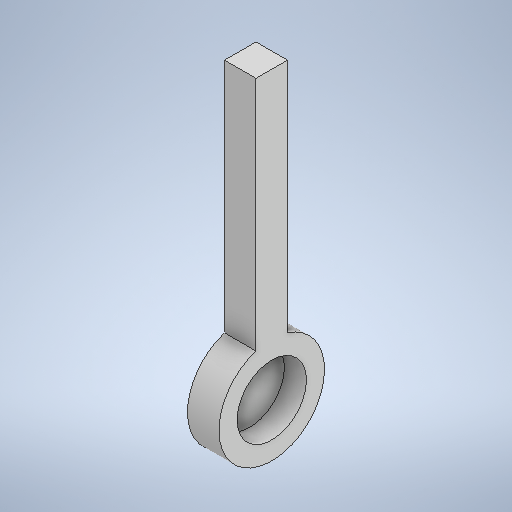
# Autodesk Inventor part: prototype3_2
Saved by Autodesk Inventor 2025.1 (Build 291241020, 241B)
## iProperties
Created: 2024-11-22
Part Number: prototype3_2
Material: Generic
Document SubType Name: Modeling
Designer: leon-
Density: 1 g/cm^3
Appearance: Default
Author: leon-
Autodesk Inventor part; units mm, degrees
ref_plane "YZ Plane" through (0, 0, 0) normal (1, 0, 0) x (0, 1, 0)
ref_plane "XZ Plane" through (0, 0, 0) normal (0, 1, 0) x (-1, 0, 0)
ref_plane "XY Plane" through (0, 0, 0) normal (0, 0, 1) x (1, 0, 0)
sketch "Sketch1" plane through (0, 0, 0) normal (0, 0, 1) x (1, 0, 0)
  line L0 (0, 0) -> (0, 16.75)
  line L1 (0, 16.75) -> (10, 16.75)
  line L2 (10, 16.75) -> (10, 11)
  line L3 (10, 11) -> (3, 11)
  line L4 (3, 11) -> (3, 0)
  line L5 (3, 0) -> (0, 0)
  point P0 (1.5, 0)
  dimension "d0" = 11
  dimension "d1" = 16.75
  dimension "d2" = 10
  dimension "d3" = 3
  constraints: 12 end point, 5 perpendicular, 1 midpoint, 1 vertical
  measures "d0" distance from line of point (1.5, 0) L3
  measures "d1" distance between parallel lines of L5 L1
  measures "d2" distance between parallel lines of L0 L2
  measures "d3" distance between parallel lines of L0 L4
revolve "Revolution1" add sketch "Sketch1" angle 360 about axis through (3, 0, 0) along (-1, 0, 0)
sketch "Sketch2" plane through (0, 0, 0) normal (0, 0, 1) x (1, 0, 0)
  line L0 (0, 16.75) -> (0, -16.75) projected
  line L1 (0, 11) -> (10, 11)
  line L2 (10, 11) -> (10, 91)
  line L3 (10, 91) -> (0, 91)
  line L4 (0, 91) -> (0, 11)
  line L5 (3, 11) -> (10, 11) projected
  line L6 (10, 16.75) -> (10, -16.75) projected
  point P0 (0, 0)
  point P1 (5, 11)
  dimension "d5" = 80
  constraints: 8 end point, 2 collinear, 2 parallel, 1 horizontal, 1 midpoint, 1 perpendicular, 1 point on line
  measures "d5" distance from line of point (5, 11) L3
extrude "Extrusion1" add sketch "Sketch2" along normal mid plane 10
body "Solid1"
